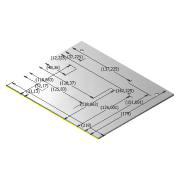
# Autodesk Inventor part: SupportsheetCDH2
Saved by Autodesk Inventor 2017 (Build 210142000, 142)
## iProperties
Created: 2016-11-08
Part Number: SupportsheetCDH2
Material: Aluminum 6061
Document SubType Name: Modeling
Designer: Jonis
Density: 2.7 g/cm^3
Appearance: Aluminum - Flat
Author: Jonis
Autodesk Inventor part; units mm, degrees
ref_plane "YZ Plane" through (0, 0, 0) normal (1, 0, 0) x (0, 1, 0)
ref_plane "XZ Plane" through (0, 0, 0) normal (0, 1, 0) x (-1, 0, 0)
ref_plane "XY Plane" through (0, 0, 0) normal (0, 0, 1) x (1, 0, 0)
sketch "Sketch1" plane through (0, 0, 0) normal (0, 0, 1) x (1, 0, 0)
  line L0 (0, 0) -> (218, 0)
  line L1 (218, 0) -> (218, 179)
  line L2 (218, 179) -> (0, 179)
  line L3 (0, 179) -> (0, 0)
  dimension "d0" = 218
  dimension "d1" = 179
  constraints: 8 end point, 2 parallel, 1 horizontal, 1 perpendicular
  measures "d0" distance of L2.end L1.end
  measures "d1" distance of L1.end L0.end
extrude "Extrusion1" add sketch "Sketch1" along normal blind 3
sketch "Sketch2" plane through (0, 0, 3) normal (0, 0, 1) x (1, 0, 0)
  line L0 (0, 179) -> (0, 0) projected
  line L1 (218, 179) -> (0, 179) projected
  line L2 (218, 0) -> (218, 179) projected
  point P0 (20, 159)
  point P1 (198, 159)
  dimension "d4" = 20
  dimension "d5" = 20
  dimension "d6" = 20
  dimension "d7" = 20
  measures "d4" distance from line of L0 point (20, 159)
  measures "d5" distance from line of L1 point (20, 159)
  measures "d6" distance from line of L1 point (198, 159)
  measures "d7" distance from line of point (198, 159) L2
hole "Hole1" at (20, 159, 3) at (198, 159, 3) direction (0, 0, -1) diameter 7 end through all
sketch "Sketch5" plane through (0, 0, 0) normal (0, 0, -1) x (-1, 0, 0)
  circle A0 centre (-125.83, 33.13) radius 1.75 projected
  circle A1 centre (-52.17, 33.13) radius 1.75 projected
  circle A2 centre (-48.3599, 118.8631) radius 1.5875 projected
  circle A3 centre (-128.3699, 118.8631) radius 1.5875 projected
  circle A4 centre (-12.2249, 126.0006) radius 1.6 projected
  circle A5 centre (-162.2249, 126.0006) radius 1.6 projected
  circle A6 centre (-37.2249, 151.0006) radius 1.6 projected
  circle A7 centre (-137.2249, 151.0006) radius 1.6 projected
  line L0 (0, 0) -> (-218, 0) projected
  line L1 (0, 179) -> (0, 0) projected
  line L2 (-218, 179) -> (0, 179) projected
  dimension "d37" = 33.13
  dimension "d38" = 118.8631
  dimension "d39" = 118.8631
  dimension "d40" = 48.3599
  dimension "d41" = 128.3699
  dimension "d42" = 52.17
  dimension "d43" = 125.83
  dimension "d44" = 12.2249
  dimension "d45" = 37.2249
  dimension "d46" = 162.2249
  dimension "d47" = 137.2249
  dimension "d48" = 218
  dimension "d49" = 179
  dimension "d50" = 126.0006
  dimension "d51" = 151.0006
  measures "d37" distance from line of A1.centre L0
  measures "d38" distance from line of L0 A2.centre
  measures "d39" distance from line of L0 A3.centre
  measures "d40" distance from line of A2.centre L1
  measures "d41" distance from line of L1 A3.centre
  measures "d42" distance from line of A1.centre L1
  measures "d43" distance from line of A0.centre L1
  measures "d44" distance from line of A4.centre L1
  measures "d45" distance from line of A6.centre L1
  measures "d46" distance from line of A5.centre L1
  measures "d47" distance from line of A7.centre L1
  measures "d48" distance of L0.start L0.end
  measures "d49" distance between parallel lines of L0 L2
  measures "d50" distance from line of A5.centre L0
  measures "d51" distance from line of A7.centre L0
body "Solid1"
